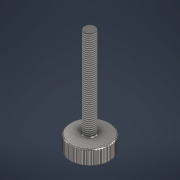
# Autodesk Inventor part: Z25_Slide_Shaft
Saved by Autodesk Inventor 2025 (Build 290162010, 162A)
## iProperties
Created: 2023-02-13
Part Number: Z25_Slide_Shaft
Material: Steel, Galvanized
Document SubType Name: Modeling
Designer: dzw04
Density: 7.85 g/cm^3
Appearance: Galvanized
Author: dzw04
Autodesk Inventor part; units mm, degrees
ref_plane "YZ Plane" through (0, 0, 0) normal (1, 0, 0) x (0, 1, 0)
ref_plane "XZ Plane" through (0, 0, 0) normal (0, 1, 0) x (-1, 0, 0)
ref_plane "XY Plane" through (0, 0, 0) normal (0, 0, 1) x (1, 0, 0)
sketch "Sketch1" plane through (0, 0, 0) normal (0, 1, 0) x (-1, 0, 0)
  circle A0 centre (0, 0.2037) radius 5.5
  point P0 (0, 0)
  dimension "d0" = 11
  constraints: 1 centre point
  measures "d0" diameter of A0
extrude "Extrusion1" add sketch "Sketch1" along normal blind 4
sketch "Sketch2" plane through (0, 4, 0.2037) normal (0, 1, 0) x (1, 0, 0)
  circle A0 centre (-0.1564, 0.0588) radius 1.5
  point P0 (0, 0.2037)
  dimension "d3" = 3
  constraints: 1 centre point
  measures "d3" diameter of A0
extrude "Extrusion2" add sketch "Sketch2" along normal blind 25
chamfer "Chamfer1" distance 0.25 angle 45 1 edges at (-1.6564, 4, 0.1449)
thread "Thread1" size "M3x0.5" class "6g" standard "ANSI Metric M Profile" full length
sketch "Sketch3" plane through (0, 0, 0.2037) normal (0, -1, 0) x (1, 0, 0)
  arc A0 (-5.4625, -0.1192) -> (-5.4625, 0.1192) centre (-5.5, 0) ccw
  arc A1 (-5.4625, -0.1192) -> (-5.4974, -0.1685) centre (-5.4474, -0.1669) ccw
  arc A2 (-5.4974, 0.1685) -> (-5.4625, 0.1192) centre (-5.4474, 0.1669) ccw
  arc A3 (-5.4974, 0.1685) -> (-5.4974, -0.1685) centre (0, 0) ccw
  dimension "d11" = 0.25
  dimension "d12" = 0.05
  constraints: 8 point on circle, 4 centre point, 2 tangent, 1 equal radius
  measures "d11" diameter of A0
  measures "d12" radius of A1
chamfer "Chamfer2" distance 0.25 angle 45 2 edges at (5.5, 0, 0.2037) (5.5, 4, 0.2037)
extrude "Extrusion3" cut sketch "Sketch3" against normal through all
pattern_circular "Circular Pattern1" count 50 over 360 about axis through (0, 0, 0.2037) along (0, 1, 0) of "Extrusion3"
body "Solid1"
